split roatry bearing v2-dup (Autodesk Fusion 360 design; units mm, degrees)
Autodesk Fusion 360 part; units mm, degrees
sketch "Sketch1" plane through (0, 0, 0) normal (0, 0, 1) x (1, 0, 0)
  circle A0 centre (0, 0) radius 15
  circle A1 centre (0, 0) radius 21
  line L0 (20.991427, 0.6) -> (49.9964, 0.6)
  line L1 (49.9964, 0.6) -> (49.9964, -0.6)
  line L2 (49.9964, -0.6) -> (20.991427, -0.6)
  line L3 (20.991427, -0.6) -> (20.991427, 0.6)
  circle A2 centre (0, 0) radius 50
  line L4 (0, 2.5) -> (0, 20)
  line L5 (-49.9964, 0.6) -> (-49.9964, -0.6)
  line L6 (-20.991427, 0.6) -> (-49.9964, 0.6)
  line L7 (-20.991427, -0.6) -> (-20.991427, 0.6)
  line L8 (-49.9964, -0.6) -> (-20.991427, -0.6)
  line L9 (-45.96104, 19.687122) -> (-46.420261, 18.578466)
  line L10 (-19.62316, 7.478744) -> (-19.16394, 8.587399)
  line L11 (-46.420261, 18.578466) -> (-19.62316, 7.478744)
  line L12 (-19.16394, 8.587399) -> (-45.96104, 19.687122)
  line L13 (19.62316, -7.478744) -> (46.420261, -18.578466)
  line L14 (46.420261, -18.578466) -> (45.96104, -19.687122)
  line L15 (19.16394, -8.587399) -> (19.62316, -7.478744)
  line L16 (45.96104, -19.687122) -> (19.16394, -8.587399)
  line L17 (-48.137522, 13.519576) -> (-48.448105, 12.360465)
  line L18 (-20.431453, 4.853426) -> (-20.12087, 6.012537)
  line L19 (-48.448105, 12.360465) -> (-20.431453, 4.853426)
  line L20 (-20.12087, 6.012537) -> (-48.137522, 13.519576)
  line L21 (20.431453, -4.853426) -> (48.448105, -12.360465)
  line L22 (48.448105, -12.360465) -> (48.137522, -13.519576)
  line L23 (20.12087, -6.012537) -> (20.431453, -4.853426)
  line L24 (48.137522, -13.519576) -> (20.12087, -6.012537)
  line L25 (-49.490358, 7.120707) -> (-49.646989, 5.930973)
  line L26 (-20.890158, 2.145064) -> (-20.733527, 3.334798)
  line L27 (-49.646989, 5.930973) -> (-20.890158, 2.145064)
  line L28 (-20.733527, 3.334798) -> (-49.490358, 7.120707)
  line L29 (20.890158, -2.145064) -> (49.646989, -5.930973)
  line L30 (49.646989, -5.930973) -> (49.490358, -7.120707)
  line L31 (20.733527, -3.334798) -> (20.890158, -2.145064)
  line L32 (49.490358, -7.120707) -> (20.733527, -3.334798)
  line L33 (-49.646989, -5.930973) -> (-49.490358, -7.120707)
  line L34 (-20.733527, -3.334798) -> (-20.890158, -2.145064)
  line L35 (-49.490358, -7.120707) -> (-20.733527, -3.334798)
  line L36 (-20.890158, -2.145064) -> (-49.646989, -5.930973)
  line L37 (20.733527, 3.334798) -> (49.490358, 7.120707)
  line L38 (49.490358, 7.120707) -> (49.646989, 5.930973)
  line L39 (20.890158, 2.145064) -> (20.733527, 3.334798)
  line L40 (49.646989, 5.930973) -> (20.890158, 2.145064)
  line L41 (-48.448105, -12.360465) -> (-48.137522, -13.519576)
  line L42 (-20.12087, -6.012537) -> (-20.431453, -4.853426)
  line L43 (-48.137522, -13.519576) -> (-20.12087, -6.012537)
  line L44 (-20.431453, -4.853426) -> (-48.448105, -12.360465)
  line L45 (20.12087, 6.012537) -> (48.137522, 13.519576)
  line L46 (48.137522, 13.519576) -> (48.448105, 12.360465)
  line L47 (20.431453, 4.853426) -> (20.12087, 6.012537)
  line L48 (48.448105, 12.360465) -> (20.431453, 4.853426)
  line L49 (-46.420261, -18.578466) -> (-45.96104, -19.687122)
  line L50 (-19.16394, -8.587399) -> (-19.62316, -7.478744)
  line L51 (-45.96104, -19.687122) -> (-19.16394, -8.587399)
  line L52 (-19.62316, -7.478744) -> (-46.420261, -18.578466)
  line L53 (19.16394, 8.587399) -> (45.96104, 19.687122)
  line L54 (45.96104, 19.687122) -> (46.420261, 18.578466)
  line L55 (19.62316, 7.478744) -> (19.16394, 8.587399)
  line L56 (46.420261, 18.578466) -> (19.62316, 7.478744)
  line L57 (-19.16394, 8.587399) -> (19.16394, 8.587399)
  line L58 (19.16394, -8.587399) -> (-19.16394, -8.587399)
  dimension "d1" = 30
  dimension "d2" = 6
  dimension "d3" = 100
  dimension "d4" = 1.2
  dimension "d6" = 45
  constraint coincident A0.centre A1.centre
  constraint horizontal L0
  constraint vertical L1
  constraint horizontal L2
  constraint vertical L3
  constraint concentric A1 A2
  constraint coincident L0.end A2
  constraint symmetric L0.end L4 L5.start
  constraint symmetric L1.end L4 L5.end
  measures "d1" diameter of A0
  measures "d2" distance of A0 A1
  measures "d3" diameter of A2
  measures "d4" distance of L0 L2
extrude "Extrude1" add sketch "Sketch1" against normal blind 3 contours A0 L57 L58 | A0 A1 L3 L15 L23 L31 L39 L47 L55 L57 L58 | A1 L53 L54 L56 | A1 L55 | A0 A1 L7 L10 L18 L26 L34 L42 L50 L57 L58 | A1 L15 | A1 L13 L14 L16 | A1 A2 L45 L56 | A1 L10 | A1 L9 L11 L12 | A2 L54 | A1 L49 L51 L52 | A1 L50 | A1 A2 L13 L24 | A2 L14 | A1 L45 L46 L48 | A1 L47 | A1 A2 L11 L20 | A2 L9 | A1 A2 L43 L52 | A2 L49 | A1 L23 | A1 L21 L22 L24 | A1 A2 L37 L48 | A2 L46 | A1 L18 | A1 L17 L19 L20 | A1 L41 L43 L44 | A1 L42 | A1 A2 L21 L32 | A2 L22 | A1 L37 L38 L40 | A1 L39 | A1 A2 L19 L28 | A2 L17 | A1 A2 L35 L44 | A2 L41 | A1 L31 | A1 L29 L30 L32 | A1 L0 A2 L40 | A2 L38 | A1 L26 | A1 L25 L27 L28 | A1 L33 L35 L36 | A1 L34 | A1 L2 A2 L29 | A2 L30 | A1 L0 L1 L2 | A1 L3 | A1 A2 L6 L27 | A2 L25 | A1 A2 L8 L36 | A2 L33 | L1 A2 | A1 L7 | A1 L5 L6 L8 | A2 L5 picked at (0, -2.862466) picked at (16.696773, -3.096223) picked at (37.235115, 15.495458) picked at (19.421412, 7.972444) picked at (-15.552568, -6.80611) picked at (19.370381, -8.095643) picked at (37.286146, -15.372259) picked at (38.627905, 11.58601) picked at (-19.421412, 7.972444) picked at (-37.235115, 15.495458) picked at (46.217149, 19.071609) picked at (-37.286146, -15.372259) picked at (-19.421412, -7.972444) picked at (38.627905, -11.58601) picked at (46.166123, -19.194795) picked at (38.939127, 10.502734) picked at (20.295872, 5.369236) picked at (-38.627905, 11.58601) picked at (-46.217149, 19.071609) picked at (-38.627905, -11.58601) picked at (-46.166123, -19.194795) picked at (20.261358, -5.498041) picked at (38.97364, -10.373929) picked at (39.809716, 6.444937) picked at (48.276589, 13.004693) picked at (-20.295872, 5.369236) picked at (-38.939127, 10.502734) picked at (-38.97364, -10.373929) picked at (-20.295872, -5.369236) picked at (39.809716, -6.444937) picked at (48.276589, -13.004693) picked at (39.976879, 5.330306) picked at (20.823064, 2.674158) picked at (-39.809716, 6.444937) picked at (-48.311099, 12.8759) picked at (-39.245752, -9.280174) picked at (-48.276589, -13.004693) picked at (20.805658, -2.806367) picked at (39.994284, -5.198097) picked at (40.310371, 1.193589) picked at (49.578433, 6.459881) picked at (-20.823064, 2.674158) picked at (-39.976879, 5.330306) picked at (-39.994284, -5.198097) picked at (-20.823064, -2.674158) picked at (40.310371, -1.193589) picked at (49.561029, -6.592077) picked at (40.330933, 0) picked at (20.993014, 0.133343) picked at (-40.121305, 4.078182) picked at (-49.561029, 6.592077) picked at (-40.121305, -4.078182) picked at (-49.561029, -6.592077) picked at (49.997067, 0.133335) picked at (-20.993967, -0.066675) picked at (-40.330616, 0.066675) picked at (-49.997467, -0.066668)
extrude "Extrude2" add sketch "Sketch1" along normal blind 60 contours A1 L53 L54 L56 | A1 L13 L14 L16 | A1 L9 L11 L12 | A1 L49 L51 L52 | A1 L45 L46 L48 | A1 L21 L22 L24 | A1 L17 L19 L20 | A1 L41 L43 L44 | A1 L37 L38 L40 | A1 L29 L30 L32 | A1 L25 L27 L28 | A1 L33 L35 L36 | A1 L0 L1 L2 | A1 L5 L6 L8 picked at (37.235115, 15.495458) picked at (37.286146, -15.372259) picked at (-37.235115, 15.495458) picked at (-37.286146, -15.372259) picked at (38.939127, 10.502734) picked at (38.97364, -10.373929) picked at (-38.939127, 10.502734) picked at (-38.97364, -10.373929) picked at (39.976879, 5.330306) picked at (39.994284, -5.198097) picked at (-39.976879, 5.330306) picked at (-39.994284, -5.198097) picked at (40.330933, 0) picked at (-40.330616, 0.066675)
extrude "Extrude3" add sketch "Sketch1" along normal blind 5 from surface at 60 contours A1 L53 L54 L56 | A1 L13 L14 L16 | A1 A2 L45 L56 | A1 L9 L11 L12 | A1 L49 L51 L52 | A1 A2 L13 L24 | A1 L45 L46 L48 | A1 A2 L11 L20 | A1 A2 L43 L52 | A1 L21 L22 L24 | A1 A2 L37 L48 | A1 L17 L19 L20 | A1 L41 L43 L44 | A1 A2 L21 L32 | A1 L37 L38 L40 | A1 A2 L19 L28 | A1 A2 L35 L44 | A1 L29 L30 L32 | A1 L0 A2 L40 | A1 L25 L27 L28 | A1 L33 L35 L36 | A1 L2 A2 L29 | A1 L0 L1 L2 | A1 A2 L6 L27 | A1 A2 L8 L36 | A1 L5 L6 L8 picked at (37.235115, 15.495458) picked at (37.286146, -15.372259) picked at (38.627905, 11.58601) picked at (-37.235115, 15.495458) picked at (-37.286146, -15.372259) picked at (38.627905, -11.58601) picked at (38.939127, 10.502734) picked at (-38.627905, 11.58601) picked at (-38.627905, -11.58601) picked at (38.97364, -10.373929) picked at (39.809716, 6.444937) picked at (-38.939127, 10.502734) picked at (-38.97364, -10.373929) picked at (39.809716, -6.444937) picked at (39.976879, 5.330306) picked at (-39.809716, 6.444937) picked at (-39.245752, -9.280174) picked at (39.994284, -5.198097) picked at (40.310371, 1.193589) picked at (-39.976879, 5.330306) picked at (-39.994284, -5.198097) picked at (40.310371, -1.193589) picked at (40.330933, 0) picked at (-40.121305, 4.078182) picked at (-40.121305, -4.078182) picked at (-40.330616, 0.066675)
sketch "Sketch2" plane through (0, 0, 65) normal (0, 0, 1) x (-1, 0, 0)
  arc A0 (19.16394, -8.587399) -> (19.16394, 8.587399) centre (0, 0) ccw
  line L0 (19.16394, -8.587399) -> (45.96104, -19.687122)
  line L1 (45.96104, -19.687122) -> (46.420261, -18.578466)
  arc A1 (46.420261, -18.578466) -> (48.137522, -13.519576) centre (0, 0) ccw
  line L2 (48.137522, -13.519576) -> (48.448105, -12.360465)
  arc A2 (48.448105, -12.360465) -> (49.490358, -7.120707) centre (0, 0) ccw
  line L3 (49.490358, -7.120707) -> (49.646989, -5.930973)
  arc A3 (49.646989, -5.930973) -> (49.9964, -0.6) centre (0, 0) ccw
  line L4 (49.9964, -0.6) -> (49.9964, 0.6)
  arc A4 (49.9964, 0.6) -> (49.646989, 5.930973) centre (0, 0) ccw
  line L5 (49.646989, 5.930973) -> (49.490358, 7.120707)
  arc A5 (49.490358, 7.120707) -> (48.448105, 12.360465) centre (0, 0) ccw
  line L6 (48.448105, 12.360465) -> (48.137522, 13.519576)
  arc A6 (48.137522, 13.519576) -> (46.420261, 18.578466) centre (0, 0) ccw
  line L7 (46.420261, 18.578466) -> (45.96104, 19.687122)
  line L8 (45.96104, 19.687122) -> (19.16394, 8.587399)
  line L9 (-45.96104, 19.687122) -> (-46.420261, 18.578466)
  arc A7 (-46.420261, 18.578466) -> (-48.137522, 13.519576) centre (0, 0) ccw
  line L10 (-48.137522, 13.519576) -> (-48.448105, 12.360465)
  arc A8 (-48.448105, 12.360465) -> (-49.490358, 7.120707) centre (0, 0) ccw
  line L11 (-49.490358, 7.120707) -> (-49.646989, 5.930973)
  arc A9 (-49.646989, 5.930973) -> (-49.9964, 0.6) centre (0, 0) ccw
  line L12 (-49.9964, 0.6) -> (-49.9964, -0.6)
  arc A10 (-49.9964, -0.6) -> (-49.646989, -5.930973) centre (0, 0) ccw
  line L13 (-49.646989, -5.930973) -> (-49.490358, -7.120707)
  arc A11 (-49.490358, -7.120707) -> (-48.448105, -12.360465) centre (0, 0) ccw
  line L14 (-48.448105, -12.360465) -> (-48.137522, -13.519576)
  arc A12 (-48.137522, -13.519576) -> (-46.420261, -18.578466) centre (0, 0) ccw
  line L15 (-46.420261, -18.578466) -> (-45.96104, -19.687122)
  line L16 (-45.96104, -19.687122) -> (-19.16394, -8.587399)
  arc A13 (-19.16394, -8.587399) -> (-19.16394, 8.587399) centre (0, 0) cw
  line L17 (-19.16394, 8.587399) -> (-45.96104, 19.687122)
  line L18 (19.16394, -8.587399) -> (-19.16394, -8.587399)
  line L19 (-19.16394, -8.587399) -> (-19.16394, 8.587399)
  line L20 (-19.16394, 8.587399) -> (19.16394, 8.587399)
  line L21 (19.16394, 8.587399) -> (19.16394, -8.587399)
  constraint horizontal L18
  constraint vertical L19
  constraint horizontal L20
  constraint vertical L21
extrude "Extrude4" add sketch "Sketch2" along normal blind 3
chamfer "Chamfer1" distance 2.943 angle 45 2 edges at (-21, 0, 65) (21, 0, 65)
